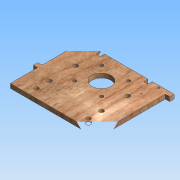
# Autodesk Inventor part: holder_plate
Saved by Autodesk Inventor 2015 (Build 190159000, 159)
## iProperties
Created: 2013-12-24
Part Number: holder_plate
Material: Wood (Birch)
Document SubType Name: Modeling
Designer: aoki
Density: 1 g/cm^3
Appearance: Birch - Natural Polished
Author: aoki
Autodesk Inventor part; units mm, degrees
ref_plane "YZ Plane" through (0, 0, 0) normal (1, 0, 0) x (0, 1, 0)
ref_plane "XZ Plane" through (0, 0, 0) normal (0, 1, 0) x (-1, 0, 0)
ref_plane "XY Plane" through (0, 0, 0) normal (0, 0, 1) x (1, 0, 0)
sketch "Block1" plane through (0, 0, 0) normal (0, 0, 1) x (1, 0, 0)
  line L0 (-30.1, 34.1) -> (-9.9, 34.1)
  line L1 (-9.9, 34.1) -> (-9.9, 25.1)
  line L2 (-9.9, 25.1) -> (9.9, 25.1)
  line L3 (9.9, 25.1) -> (9.9, 34.1)
  line L4 (9.9, 34.1) -> (30.1, 34.1)
  line L5 (30.1, 34.1) -> (30.1, 25.1)
  line L6 (30.1, 25.1) -> (50.1, 25.1)
  line L7 (50.1, 25.1) -> (50.1, 16.5667)
  line L8 (50.1, 16.5667) -> (41.1, 16.5667)
  line L9 (41.1, 16.5667) -> (41.1, 6.7667)
  line L10 (41.1, 6.7667) -> (50.1, 6.7667)
  line L11 (50.1, 6.7667) -> (50.1, -6.7667)
  line L12 (50.1, -6.7667) -> (41.1, -6.7667)
  line L13 (41.1, -6.7667) -> (41.1, -16.5667)
  line L14 (41.1, -16.5667) -> (50.1, -16.5667)
  line L15 (50.1, -16.5667) -> (50.1, -25.1)
  line L16 (50.1, -25.1) -> (30.1, -25.1)
  line L17 (30.1, -25.1) -> (30.1, -34.1)
  line L18 (30.1, -34.1) -> (9.9, -34.1)
  line L19 (9.9, -34.1) -> (9.9, -25.1)
  line L20 (9.9, -25.1) -> (-9.9, -25.1)
  line L21 (-9.9, -25.1) -> (-9.9, -34.1)
  line L22 (-9.9, -34.1) -> (-30.1, -34.1)
  line L23 (-30.1, -34.1) -> (-30.1, -25.1)
  line L24 (-30.1, -25.1) -> (-50.1, -25.1)
  line L25 (-50.1, -25.1) -> (-50.1, -16.5667)
  line L26 (-50.1, -16.5667) -> (-41.1, -16.5667)
  line L27 (-41.1, -16.5667) -> (-41.1, -6.7667)
  line L28 (-41.1, -6.7667) -> (-50.1, -6.7667)
  line L29 (-50.1, -6.7667) -> (-50.1, 6.7667)
  line L30 (-50.1, 6.7667) -> (-41.1, 6.7667)
  line L31 (-41.1, 6.7667) -> (-41.1, 16.5667)
  line L32 (-41.1, 16.5667) -> (-50.1, 16.5667)
  line L33 (-50.1, 16.5667) -> (-50.1, 25.1)
  line L34 (-50.1, 25.1) -> (-30.1, 25.1)
  line L35 (-30.1, 25.1) -> (-30.1, 34.1)
  circle A0 centre (-30, 0) radius 4.6
  circle A1 centre (-15.5, 15.5) radius 2.1
  circle A2 centre (-15.5, -15.5) radius 2.1
  circle A3 centre (0, 0) radius 11.1
  circle A4 centre (15.5, 15.5) radius 2.1
  circle A5 centre (30, 0) radius 4.6
  circle A6 centre (15.5, -15.5) radius 2.1
  point P0 (0, 0)
sketch "Block2" plane through (0, 0, 0) normal (0, 0, 1) x (1, 0, 0)
  line L0 (9.8, 34.2) -> (30.2, 34.2)
  line L1 (30.2, 34.2) -> (30.2, 25.2)
  line L2 (30.2, 25.2) -> (50.2, 25.2)
  line L3 (50.2, 25.2) -> (50.2, 16.4667)
  line L4 (50.2, 16.4667) -> (41.2, 16.4667)
  line L5 (41.2, 16.4667) -> (41.2, 6.8667)
  line L6 (41.2, 6.8667) -> (50.2, 6.8667)
  line L7 (50.2, 6.8667) -> (50.2, -6.8667)
  line L8 (50.2, -6.8667) -> (41.2, -6.8667)
  line L9 (41.2, -6.8667) -> (41.2, -16.4667)
  line L10 (41.2, -16.4667) -> (50.2, -16.4667)
  line L11 (50.2, -16.4667) -> (50.2, -25.2)
  line L12 (50.2, -25.2) -> (30.2, -25.2)
  line L13 (30.2, -25.2) -> (30.2, -34.2)
  line L14 (30.2, -34.2) -> (9.8, -34.2)
  line L15 (9.8, -34.2) -> (9.8, -25.2)
  line L16 (9.8, -25.2) -> (-9.8, -25.2)
  line L17 (-9.8, -25.2) -> (-9.8, -34.2)
  line L18 (-9.8, -34.2) -> (-30.2, -34.2)
  line L19 (-30.2, -34.2) -> (-30.2, -25.2)
  line L20 (-30.2, -25.2) -> (-50.2, -25.2)
  line L21 (-50.2, -25.2) -> (-50.2, -16.4667)
  line L22 (-50.2, -16.4667) -> (-41.2, -16.4667)
  line L23 (-41.2, -16.4667) -> (-41.2, -6.8667)
  line L24 (-41.2, -6.8667) -> (-50.2, -6.8667)
  line L25 (-50.2, -6.8667) -> (-50.2, 6.8667)
  line L26 (-50.2, 6.8667) -> (-41.2, 6.8667)
  line L27 (-41.2, 6.8667) -> (-41.2, 16.4667)
  line L28 (-41.2, 16.4667) -> (-50.2, 16.4667)
  line L29 (-50.2, 16.4667) -> (-50.2, 25.2)
  line L30 (-50.2, 25.2) -> (-30.2, 25.2)
  line L31 (-30.2, 25.2) -> (-30.2, 34.2)
  line L32 (-30.2, 34.2) -> (-9.8, 34.2)
  line L33 (-9.8, 34.2) -> (-9.8, 25.2)
  line L34 (-9.8, 25.2) -> (9.8, 25.2)
  line L35 (9.8, 25.2) -> (9.8, 34.2)
  circle A0 centre (-15.5, 15.5) radius 2.2
  circle A1 centre (15.5, 15.5) radius 2.2
  circle A2 centre (30, 0) radius 4.7
  circle A3 centre (15.5, -15.5) radius 2.2
  circle A4 centre (-15.5, -15.5) radius 2.2
  circle A5 centre (-30, 0) radius 4.7
  circle A6 centre (0, 0) radius 11.2
  point P0 (0, 0)
sketch "Block3" plane through (0, 0, 0) normal (0, 0, 1) x (1, 0, 0)
  line L0 (9.9, 34.1) -> (30.1, 34.1)
  line L1 (30.1, 34.1) -> (30.1, 25.1)
  line L2 (30.1, 25.1) -> (50.1, 25.1)
  line L3 (50.1, 25.1) -> (50.1, 16.5667)
  line L4 (50.1, 16.5667) -> (41.1, 16.5667)
  line L5 (41.1, 16.5667) -> (41.1, 6.7667)
  line L6 (41.1, 6.7667) -> (50.1, 6.7667)
  line L7 (50.1, 6.7667) -> (50.1, -6.7667)
  line L8 (50.1, -6.7667) -> (41.1, -6.7667)
  line L9 (41.1, -6.7667) -> (41.1, -16.5667)
  line L10 (41.1, -16.5667) -> (50.1, -16.5667)
  line L11 (50.1, -16.5667) -> (50.1, -25.1)
  line L12 (50.1, -25.1) -> (30.1, -25.1)
  line L13 (30.1, -25.1) -> (30.1, -34.1)
  line L14 (30.1, -34.1) -> (9.9, -34.1)
  line L15 (9.9, -34.1) -> (9.9, -25.1)
  line L16 (9.9, -25.1) -> (-9.9, -25.1)
  line L17 (-9.9, -25.1) -> (-9.9, -34.1)
  line L18 (-9.9, -34.1) -> (-30.1, -34.1)
  line L19 (-30.1, -34.1) -> (-30.1, -25.1)
  line L20 (-30.1, -25.1) -> (-50.1, -25.1)
  line L21 (-50.1, -25.1) -> (-50.1, -16.5667)
  line L22 (-50.1, -16.5667) -> (-41.1, -16.5667)
  line L23 (-41.1, -16.5667) -> (-41.1, -6.7667)
  line L24 (-41.1, -6.7667) -> (-50.1, -6.7667)
  line L25 (-50.1, -6.7667) -> (-50.1, 6.7667)
  line L26 (-50.1, 6.7667) -> (-41.1, 6.7667)
  line L27 (-41.1, 6.7667) -> (-41.1, 16.5667)
  line L28 (-41.1, 16.5667) -> (-50.1, 16.5667)
  line L29 (-50.1, 16.5667) -> (-50.1, 25.1)
  line L30 (-50.1, 25.1) -> (-30.1, 25.1)
  line L31 (-30.1, 25.1) -> (-30.1, 34.1)
  line L32 (-30.1, 34.1) -> (-9.9, 34.1)
  line L33 (-9.9, 34.1) -> (-9.9, 25.1)
  line L34 (-9.9, 25.1) -> (9.9, 25.1)
  line L35 (9.9, 25.1) -> (9.9, 34.1)
  circle A0 centre (-15.5, 15.5) radius 2.1
  circle A1 centre (15.5, 15.5) radius 2.1
  circle A2 centre (30, 0) radius 4.6
  circle A3 centre (15.5, -15.5) radius 2.1
  circle A4 centre (-15.5, -15.5) radius 2.1
  circle A5 centre (-30, 0) radius 4.6
  circle A6 centre (0, 0) radius 11.1
  point P0 (0, 0)
sketch "Block4" plane through (0, 0, 0) normal (0, 0, 1) x (1, 0, 0)
  line L0 (-30.08, 30.58) -> (-9.92, 30.58)
  line L1 (-9.92, 30.58) -> (-9.92, 25.08)
  line L2 (-9.92, 25.08) -> (9.92, 25.08)
  line L3 (9.92, 25.08) -> (9.92, 30.58)
  line L4 (9.92, 30.58) -> (30.08, 30.58)
  line L5 (30.08, 30.58) -> (30.08, 25.08)
  line L6 (30.08, 25.08) -> (50.08, 25.08)
  line L7 (50.08, 25.08) -> (50.08, 16.5867)
  line L8 (50.08, 16.5867) -> (44.58, 16.5867)
  line L9 (44.58, 16.5867) -> (44.58, 6.7467)
  line L10 (44.58, 6.7467) -> (50.08, 6.7467)
  line L11 (50.08, 6.7467) -> (50.08, -6.7467)
  line L12 (50.08, -6.7467) -> (44.58, -6.7467)
  line L13 (44.58, -6.7467) -> (44.58, -16.5867)
  line L14 (44.58, -16.5867) -> (50.08, -16.5867)
  line L15 (50.08, -16.5867) -> (50.08, -25.08)
  line L16 (50.08, -25.08) -> (30.08, -25.08)
  line L17 (30.08, -25.08) -> (30.08, -30.58)
  line L18 (30.08, -30.58) -> (9.92, -30.58)
  line L19 (9.92, -30.58) -> (9.92, -25.08)
  line L20 (9.92, -25.08) -> (-9.92, -25.08)
  line L21 (-9.92, -25.08) -> (-9.92, -30.58)
  line L22 (-9.92, -30.58) -> (-30.08, -30.58)
  line L23 (-30.08, -30.58) -> (-30.08, -25.08)
  line L24 (-30.08, -25.08) -> (-50.08, -25.08)
  line L25 (-50.08, -25.08) -> (-50.08, -16.5867)
  line L26 (-50.08, -16.5867) -> (-44.58, -16.5867)
  line L27 (-44.58, -16.5867) -> (-44.58, -6.7467)
  line L28 (-44.58, -6.7467) -> (-50.08, -6.7467)
  line L29 (-50.08, -6.7467) -> (-50.08, 6.7467)
  line L30 (-50.08, 6.7467) -> (-44.58, 6.7467)
  line L31 (-44.58, 6.7467) -> (-44.58, 16.5867)
  line L32 (-44.58, 16.5867) -> (-50.08, 16.5867)
  line L33 (-50.08, 16.5867) -> (-50.08, 25.08)
  line L34 (-50.08, 25.08) -> (-30.08, 25.08)
  line L35 (-30.08, 25.08) -> (-30.08, 30.58)
  circle A0 centre (-30, 0) radius 4.88
  circle A1 centre (30, 0) radius 4.88
  circle A2 centre (15.5, 15.5) radius 2.08
  circle A3 centre (0, 0) radius 11.08
  circle A4 centre (-15.5, 15.5) radius 2.08
  circle A5 centre (-15.5, -15.5) radius 2.08
  circle A6 centre (15.5, -15.5) radius 2.08
  point P0 (0, 0)
sketch "Sketch10" plane through (0, 0, 0) normal (0, 0, 1) x (1, 0, 0)
  line L0 (50, -25) -> (-50, -25)
  line L1 (-50, -25) -> (-50, 25)
  line L2 (-50, 25) -> (50, 25)
  line L3 (50, 25) -> (50, -25)
  line L4 (50, -25) -> (-50, 25) construction
  line L5 (-50, -25) -> (50, 25) construction
  line L6 (-50, 25) -> (50, 25)
  line L7 (50, 25) -> (50, 28.5)
  line L8 (50, 28.5) -> (-50, 28.5)
  line L9 (-50, 28.5) -> (-50, 25)
  line L10 (69, -18.5) -> (74, -18.5) projected
  point P0 (0, 0)
  dimension "d21" = 100
  dimension "d22" = 50
  dimension "d202" = 47
  constraints: 20 end point, 4 parallel, 2 horizontal, 2 midpoint, 2 perpendicular
  measures "d21" distance of L1.end L2.end
  measures "d22" distance of L0.end L1.end
  measures "d202" distance between parallel lines of L10 L8
extrude "Extrusion2" add sketch "Sketch10" against normal blind 5 contours L0 L1 L2 L3
sketch "Sketch13" plane through (0, 0, 0) normal (0, 0, 1) x (1, 0, 0)
  line L0 (0, -35) -> (0, 35) projected
  line L1 (-70, 0) -> (70, 0) projected
  point P0 (-15.5, 15.5)
  point P1 (15.5, 15.5)
  point P2 (-15.5, -15.5)
  point P3 (15.5, -15.5)
  dimension "d43" = 31
  dimension "d44" = 31
  constraints: 3 symmetric about line
  measures "d43" distance of point (15.5, 15.5) point (-15.5, 15.5)
  measures "d44" distance of point (-15.5, -15.5) point (-15.5, 15.5)
hole "Hole4" at (-15.5, 15.5, 0) at (15.5, 15.5, 0) at (-15.5, -15.5, 0) at (15.5, -15.5, 0) direction (0, 0, -1) diameter 4 end through all
sketch "Sketch16" plane through (0, 0, -5) normal (0, 0, -1) x (-1, 0, 0)
  line L0 (0, -35) -> (0, 35) projected
  point P0 (0, 0)
  point P1 (-30, 0)
  point P2 (30, 0)
  dimension "d52" = 60
  constraints: 1 symmetric about line
  measures "d52" distance of point (30, 0) point (-30, 0)
hole "Hole5" at (30, 0, -5) at (-30, 0, -5) direction (0, 0, 1) diameter 5.2 end through all
sketch "Sketch17" plane through (0, 0, -5) normal (0, 0, -1) x (-1, 0, 0)
  point P0 (0, 0)
  point P1 (0, 0)
  constraints: 1 coincident
hole "Hole8" at (0, 0, -5) direction (0, 0, 1) diameter 22 end through all
sketch "Sketch44" plane through (0, 0, 0) normal (0, 0, 1) x (1, 0, 0)
  circle A0 centre (0, 0) radius 11 projected
  circle A1 centre (30, 0) radius 2.6 projected
  circle A2 centre (-30, 0) radius 2.6 projected
  circle A3 centre (-15.5, -15.5) radius 2 projected
  circle A4 centre (-15.5, 15.5) radius 2 projected
  circle A5 centre (15.5, 15.5) radius 2 projected
  circle A6 centre (15.5, -15.5) radius 2 projected
  line L0 (50, -25) -> (-50, -25) projected
  line L1 (50, 25) -> (50, -25) projected
  line L2 (-50, 25) -> (50, 25) projected
  line L3 (-50, -25) -> (-50, 25) projected
  line L4 (-50, -25) -> (50, -25)
  line L5 (50, -25) -> (50, -55)
  line L6 (50, -55) -> (-50, -55)
  line L7 (-50, -55) -> (-50, -25)
  circle A7 centre (30, -45) radius 2.5
  line L8 (50, 25) -> (50, -25) projected
  circle A8 centre (-30, -45) radius 2.5
  line L9 (-70, 0) -> (70, 0) projected
  line L10 (0, -71) -> (0, 41) projected
  circle A9 centre (30, -30) radius 2.5
  circle A10 centre (-30, -30) radius 2.5
  dimension "d176" = 30
  dimension "d179" = 5
  dimension "d184" = 5
  dimension "d185" = 10
  dimension "d189" = 60
  dimension "d190" = 30
  dimension "d191" = 10
  dimension "d192" = 5
  dimension "d193" = 15
  dimension "d196" = 5
  constraints: 8 end point, 4 centre point, 2 parallel, 1 collinear, 1 horizontal, 1 perpendicular
  measures "d176" distance of L6.end L0.end
  measures "d179" diameter of A7
  measures "d184" diameter of A8
  measures "d185" distance from line of L6 A8.centre
  measures "d189" distance of A8.centre A7.centre
  measures "d190" distance from line of L10 A7.centre
  measures "d191" distance from line of L6 A7.centre
  measures "d192" diameter of A9
  measures "d193" distance of A7.centre A9.centre
  measures "d196" diameter of A10
extrude "Extrusion11" add sketch "Sketch44" against normal blind 5 contours L10 L6 L7 L0 | L0 L5 L6 L10
sketch "Sketch45" plane through (0, 0, 0) normal (0, 0, 1) x (1, 0, 0)
  circle A0 centre (30, -45) radius 2.5 projected
  circle A1 centre (-30, -45) radius 2.5 projected
  circle A2 centre (30, -30) radius 2.5 projected
  circle A3 centre (-30, -30) radius 2.5 projected
  circle A4 centre (0, 0) radius 11 projected
  circle A5 centre (30, 0) radius 2.6 projected
  circle A6 centre (-30, 0) radius 2.6 projected
  circle A7 centre (-15.5, -15.5) radius 2 projected
  circle A8 centre (-15.5, 15.5) radius 2 projected
  circle A9 centre (15.5, 15.5) radius 2 projected
  circle A10 centre (15.5, -15.5) radius 2 projected
  line L0 (50, 25) -> (50, -55) projected
  line L1 (-50, 25) -> (50, 25) projected
  line L2 (-50, 25) -> (-50, -55) projected
  line L3 (-50, -55) -> (50, -55) projected
  line L4 (-50, 28.5) -> (50, 28.5) projected
  line L5 (-50, 25) -> (50, 25)
  line L6 (50, 25) -> (50, 28.5)
  line L7 (50, 28.5) -> (-50, 28.5)
  line L8 (-50, 28.5) -> (-50, 25)
  constraints: 8 end point, 2 parallel, 1 horizontal, 1 perpendicular
extrude "Extrusion12" add sketch "Sketch45" against normal blind 5 contours L1 L8 L4 L6
sketch "Sketch46" plane through (0, 0, 0) normal (0, 0, 1) x (1, 0, 0)
  line L0 (-30, 28.5) -> (-25, 28.5)
  line L1 (-25, 28.5) -> (-25, 23.5)
  line L2 (-25, 23.5) -> (-30, 23.5)
  line L3 (-30, 23.5) -> (-30, 28.5)
  line L4 (-30, 28.5) -> (-25, 23.5) construction
  line L5 (-25, 28.5) -> (-30, 23.5) construction
  line L6 (-50, 28.5) -> (-50, -55) projected
  line L7 (50, 28.5) -> (-50, 28.5) projected
  line L8 (25, 23.5) -> (30, 23.5)
  line L9 (30, 23.5) -> (30, 28.5)
  line L10 (30, 28.5) -> (25, 28.5)
  line L11 (25, 28.5) -> (25, 23.5)
  line L12 (25, 23.5) -> (30, 28.5) construction
  line L13 (30, 23.5) -> (25, 28.5) construction
  line L14 (50, -55) -> (50, 28.5) projected
  point P0 (0, 0)
  point P1 (-27.5, 26)
  point P2 (27.5, 26)
  dimension "d203" = 5
  dimension "d204" = 5
  dimension "d205" = 20
  dimension "d206" = 5
  dimension "d207" = 5
  dimension "d208" = 20
  constraints: 24 end point, 4 midpoint, 4 parallel, 2 collinear, 2 horizontal, 2 perpendicular
  measures "d203" distance of L1.end L2.end
  measures "d204" distance of L0.end L1.end
  measures "d205" distance between parallel lines of L6 L3
  measures "d206" distance of L10.end L9.end
  measures "d207" distance of L9.end L8.end
  measures "d208" distance between parallel lines of L14 L9
extrude "Extrusion13" cut sketch "Sketch46" against normal through all
sketch "Sketch47" plane through (0, 0, 0) normal (0, 0, 1) x (1, 0, 0)
  circle A0 centre (-40, 26) radius 1
  line L0 (-30, 28.5) -> (-50, 28.5) projected
  line L1 (-50, 28.5) -> (-50, -55) projected
  point P0 (0, 0)
  dimension "d211" = 2
  dimension "d212" = 2.5
  dimension "d213" = 10
  constraints: 1 centre point
  measures "d211" diameter of A0
  measures "d212" distance from line of L0 A0.centre
  measures "d213" distance from line of L1 A0.centre
sketch "Sketch48" plane through (0, 0, 0) normal (0, 0, 1) x (1, 0, 0)
  circle A0 centre (40, 26) radius 1
  line L0 (50, -55) -> (50, 28.5) projected
  line L1 (50, 28.5) -> (30, 28.5) projected
  point P0 (0, 0)
  dimension "d214" = 2
  dimension "d215" = 10
  dimension "d216" = 2.5
  constraints: 1 centre point
  measures "d214" diameter of A0
  measures "d215" distance from line of L0 A0.centre
  measures "d216" distance from line of L1 A0.centre
extrude "Extrusion14" cut sketch "Sketch48" against normal through all
extrude "Extrusion15" cut sketch "Sketch47" against normal through all
sketch "Sketch49" plane through (0, 0, 0) normal (0, 0, 1) x (1, 0, 0)
  line L0 (-55, 28.5) -> (-50, 28.5)
  line L1 (-50, 28.5) -> (-50, 23.5)
  line L2 (-50, 23.5) -> (-55, 23.5)
  line L3 (-55, 23.5) -> (-55, 28.5)
  line L4 (-50, 28.5) -> (-50, -55) projected
  line L5 (-30, 28.5) -> (-50, 28.5) projected
  line L6 (50, 28.5) -> (55, 28.5)
  line L7 (55, 28.5) -> (55, 23.5)
  line L8 (55, 23.5) -> (50, 23.5)
  line L9 (50, 23.5) -> (50, 28.5)
  line L10 (50, -55) -> (50, 28.5) projected
  line L11 (50, 28.5) -> (30, 28.5) projected
  point P0 (0, 0)
  dimension "d221" = 5
  dimension "d222" = 5
  dimension "d223" = 5
  dimension "d224" = 5
  constraints: 16 end point, 4 collinear, 4 parallel, 2 horizontal, 2 perpendicular
  measures "d221" distance of L1.end L2.end
  measures "d222" distance of L0.end L1.end
  measures "d223" distance of L7.end L8.end
  measures "d224" distance of L6.end L7.end
extrude "Extrusion16" add sketch "Sketch49" against normal blind 5
sketch "Sketch50" plane through (0, 0, 0) normal (0, 0, 1) x (1, 0, 0)
  line L0 (-50, -18.5) -> (-55, -18.5)
  line L1 (-55, -18.5) -> (-55, -23.5)
  line L2 (-55, -23.5) -> (-50, -23.5)
  line L3 (-50, -23.5) -> (-50, -18.5)
  line L4 (-30, 28.5) -> (-55, 28.5) projected
  line L5 (-50, 23.5) -> (-50, -55) projected
  point P0 (0, 0)
  dimension "d227" = 5
  dimension "d228" = 5
  dimension "d229" = 47
  constraints: 8 end point, 2 parallel, 1 collinear, 1 horizontal, 1 perpendicular
  measures "d227" distance of L2.end L1.end
  measures "d228" distance of L1.end L0.end
  measures "d229" distance between parallel lines of L4 L0
extrude "Extrusion17" add sketch "Sketch50" against normal blind 5
body "Solid2"
